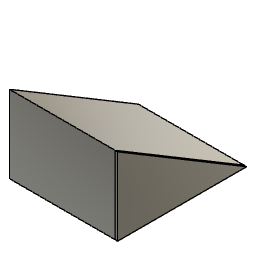
clamp (Autodesk Fusion 360 design; units mm, degrees)
Autodesk Fusion 360 part; units mm, degrees
sketch "Sketch8" plane through (0, 0, 0) normal (1, 0, 0) x (0, 1, 0)
  line L0 (0, 0) -> (0, -30)
  line L1 (0, -30) -> (50, -30)
  line L2 (50, -30) -> (0, 0)
  line L3 (0, -30, 50) -> (50, -30, 50)
  line L4 (50, -30, 50) -> (0, 0, 50)
  line L5 (0, 0, 50) -> (0, -30, 50)
  dimension "d23" = 30
  dimension "d24" = 50
  dimension "d28" = 30
  dimension "d29" = 50
  constraint coincident L0.start L2.end
  constraint vertical L0
  constraint perpendicular L0 L1
  measures "d23" distance of L0.start L0.end
  measures "d24" distance of L0.end L1.end
  measures "d28" distance of L0.end L0.start
  measures "d29" distance of L1.end L0.end
extrude "Extrude6" add sketch "Sketch8" along normal blind 40 thin wall 1 inside makes body 1
sketch "Sketch9" plane through (0, 0, 0) normal (1, 0, 0) x (0, 1, 0)
  line L0 (0, 0) -> (0, -30)
  line L1 (0, -30) -> (50, -30)
  line L2 (50, -30) -> (0, 0)
  constraint coincident L0.start L2.end
  constraint vertical L0
  constraint perpendicular L0 L1
extrude "Extrude7" add sketch "Sketch9" against normal blind 1 separate body makes body 2
move_body "Move1" bodies 2 to x (1, 0, 0) y (0, 1, 0) z (0, 0, 1) at (41, 0, 0)
extrude "Extrude8" add sketch "Sketch8" against normal blind 1 bodies 1
move_body "Move2" bodies 2 1 to x (1, 0, 0) y (0, 1, 0) z (0, 0, 1) at (-5, -10, 0)
